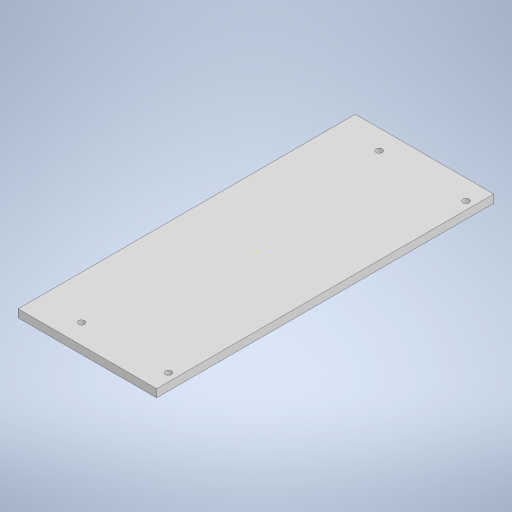
# Autodesk Inventor part: Деталь4
Saved by Autodesk Inventor 2023.1 (Build 271208000, 208)
## iProperties
Created: 2026-02-21
Part Number: Деталь4
Material: Типовые
Document SubType Name: Modeling
Designer: DELL
Density: 1 g/cm^3
Appearance: По умолчанию
Author: DELL
Autodesk Inventor part; units mm, degrees
ref_plane "YZ Plane" through (0, 0, 0) normal (1, 0, 0) x (0, 1, 0)
ref_plane "XZ Plane" through (0, 0, 0) normal (0, 1, 0) x (-1, 0, 0)
ref_plane "XY Plane" through (0, 0, 0) normal (0, 0, 1) x (1, 0, 0)
sketch "Эскиз1" plane through (0, 0, 0) normal (0, 1, 0) x (-1, 0, 0)
  line L0 (-35, 85.25) -> (35, 85.25)
  line L1 (35, 85.25) -> (35, -85.25)
  line L2 (35, -85.25) -> (-35, -85.25)
  line L3 (-35, -85.25) -> (-35, 85.25)
  line L4 (-35, 85.25) -> (35, -85.25) construction
  line L5 (35, 85.25) -> (-35, -85.25) construction
  circle A0 centre (13, 75.25) radius 1.6
  circle A1 centre (-31, 75.25) radius 1.6
  line L6 (35, 0) -> (0, 0) construction
  line L7 (-35, -85.25) -> (35, 85.25) construction
  circle A2 centre (13, -75.25) radius 1.6
  circle A3 centre (-31, -75.25) radius 1.6
  dimension "d0" = 170.5
  dimension "d1" = 70
  dimension "d2" = 3.2
  dimension "d3" = 22
  dimension "d4" = 10
  dimension "d5" = 3.2
  dimension "d6" = 4
  dimension "d7" = 10
  constraints: 16 end point, 4 centre point, 3 midpoint, 2 horizontal, 2 parallel, 2 symmetric about line, 1 perpendicular, 2 other
  measures "d0" distance of L2.end L0.start
  measures "d1" distance of L0.start L0.end
  measures "d2" diameter of A0
  measures "d3" distance from line of L1 A0.centre
  measures "d4" distance from line of L0 A0.centre
  measures "d5" diameter of A1
  measures "d6" distance from line of L3 A1.centre
  measures "d7" distance from line of L0 A1.centre
extrude "Выдавливание1" add sketch "Эскиз1" along normal blind 4
sketch "Эскиз2" plane through (0, 4, 0) normal (0, 1, 0) x (1, 0, 0)
  point P0 (0, 0)
